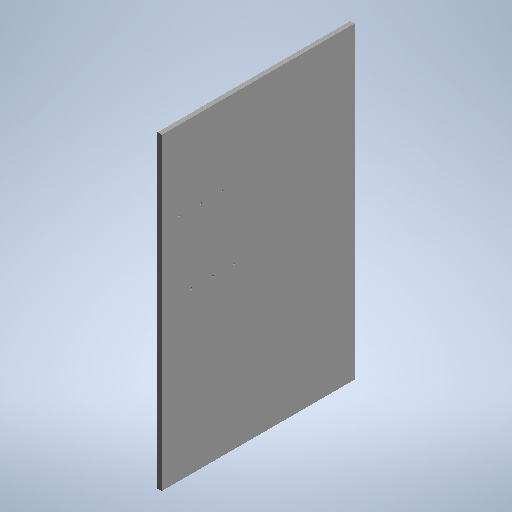
# Autodesk Inventor part: RT_ELE_MC_017_MainBackPlate
Saved by Autodesk Inventor 2025.4 (Build 294407000, 407)
## iProperties
Created: 2026-07-07
Part Number: RT_ELE_MC_017_MainBackPlate
Material: UHMW, Black
Document SubType Name: Modeling
Designer: louis
Density: 0.94 g/cm^3
Appearance: Par défaut
Mass: 1826.82 g
Surface Area: 6623.58 cm^2
Volume: 1943.43 cm^3
Author: louis
Autodesk Inventor part; units mm, degrees
ref_plane "YZ Plane" through (0, 0, 0) normal (1, 0, 0) x (0, 1, 0)
ref_plane "XZ Plane" through (0, 0, 0) normal (0, 1, 0) x (-1, 0, 0)
ref_plane "XY Plane" through (0, 0, 0) normal (0, 0, 1) x (1, 0, 0)
sketch "Sketch2" plane through (0, 0, 0) normal (1, 0, 0) x (0, 1, 0)
  line L0 (-225, 360) -> (225, 360)
  line L1 (225, 360) -> (225, -360)
  line L2 (225, -360) -> (-225, -360)
  line L3 (-225, -360) -> (-225, 360)
  line L4 (-225, 360) -> (225, -360) construction
  line L5 (225, 360) -> (-225, -360) construction
  point P0 (0, 0)
  dimension "d0" = 450
  dimension "d1" = 720
  constraints: 12 end point, 2 midpoint, 2 parallel, 1 horizontal, 1 perpendicular
  measures "d0" distance of L1.end L2.end
  measures "d1" distance of L0.end L1.end
extrude "Extrusion1" add sketch "Sketch2" along normal mid plane 10
sketch "Sketch3" plane through (5, 0, 0) normal (1, 0, 0) x (0, 0, -1)
  line L0 (360, -225) -> (360, 225) projected
  line L1 (360, 225) -> (-360, 225) projected
  line L2 (-360, 225) -> (-360, -225) projected
  line L3 (-360, -225) -> (360, -225) projected
  line L4 (-335, -200) -> (-335, 200)
  line L5 (-335, 200) -> (335, 200)
  line L6 (335, 200) -> (335, -200)
  line L7 (335, -200) -> (-335, -200)
  line L8 (-175.5, -184) -> (-175.5, -134) construction
  line L9 (-175.5, -134) -> (-175.5, -84) construction
  line L10 (-175.5, -184) -> (-14.5, -156) construction
  line L11 (-175.5, -134) -> (-14.5, -106) construction
  line L12 (-175.5, -84) -> (-14.5, -56) construction
  line L13 (-180, -190) -> (-10, -190)
  line L14 (-10, -190) -> (-10, -150)
  line L15 (-10, -150) -> (-180, -150)
  line L16 (-180, -150) -> (-180, -190)
  line L17 (-180, -190) -> (-10, -150) construction
  line L18 (-10, -190) -> (-180, -150) construction
  line L19 (-180, -140) -> (-10, -140)
  line L20 (-10, -140) -> (-10, -100)
  line L21 (-10, -100) -> (-180, -100)
  line L22 (-180, -100) -> (-180, -140)
  line L23 (-180, -140) -> (-10, -100) construction
  line L24 (-10, -140) -> (-180, -100) construction
  line L25 (-180, -90) -> (-10, -90)
  line L26 (-10, -90) -> (-10, -50)
  line L27 (-10, -50) -> (-180, -50)
  line L28 (-180, -50) -> (-180, -90)
  line L29 (-180, -90) -> (-10, -50) construction
  line L30 (-10, -90) -> (-180, -50) construction
  point P0 (0, 0)
  point P1 (-95, -170)
  point P2 (-95, -120)
  point P3 (-95, -70)
  dimension "d4" = 25
  dimension "d5" = 28
  dimension "d6" = 161
  dimension "d7" = 161
  dimension "d8" = 28
  dimension "d9" = 28
  dimension "d10" = 161
  dimension "d11" = 50
  dimension "d12" = 50
  dimension "d13" = 170
  dimension "d14" = 40
  dimension "d15" = 170
  dimension "d16" = 40
  dimension "d17" = 170
  dimension "d18" = 40
  dimension "d21" = 10
  dimension "d29" = 155
  constraints: 54 end point, 9 midpoint, 6 parallel, 3 horizontal, 3 perpendicular, 2 vertical, 3 other
  measures "d4" distance between parallel lines of L2 L4
  measures "d5" vertical distance of L10.end L8.start
  measures "d6" horizontal distance of L8.start L10.end
  measures "d7" horizontal distance of L11.end L9.start
  measures "d8" vertical distance of L11.end L9.start
  measures "d9" vertical distance of L12.end L12.start
  measures "d10" horizontal distance of L12.end L12.start
  measures "d11" distance of L8.start L9.start
  measures "d12" distance of L9.start L12.start
  measures "d13" distance of L15.end L14.end
  measures "d14" distance of L14.end L13.end
  measures "d15" distance of L21.end L21.start
  measures "d16" distance of L21.start L20.start
  measures "d17" distance of L27.end L27.start
  measures "d18" distance of L27.start L25.end
  measures "d21" distance between parallel lines of L7 L13
  measures "d29" horizontal distance of L4.start L13.start
hole "Hole1" at (5, -84, 175.5) at (5, -56, 14.5) at (5, -134, 175.5) at (5, -106, 14.5) at (5, -184, 175.5) at (5, -156, 14.5) direction (-1, 0, 0) diameter 4.5 end through all clearance for "Flat Head Machine Screw" size "M4" standard "Ansi Metric M Profile"
body "Solid1"
